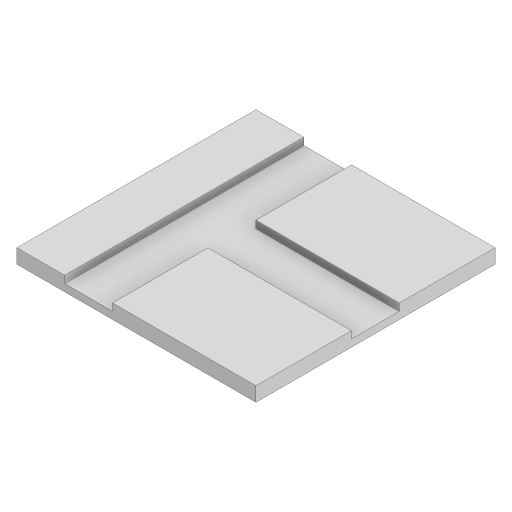
# Autodesk Inventor part: T_intersection_simple
Saved by Autodesk Inventor 2023 (Build 270158000, 158)
## iProperties
Created: 2022-07-19
Part Number: T_intersection_simple
Material: Generic
Document SubType Name: Modeling
Designer: Derm
Density: 1 g/cm^3
Appearance: Default
Author: Derm
Autodesk Inventor part; units mm, degrees
ref_plane "YZ Plane" through (0, 0, 0) normal (1, 0, 0) x (0, 1, 0)
ref_plane "XZ Plane" through (0, 0, 0) normal (0, 1, 0) x (-1, 0, 0)
ref_plane "XY Plane" through (0, 0, 0) normal (0, 0, 1) x (1, 0, 0)
sketch "Sketch1" plane through (0, 0, 0) normal (0, 1, 0) x (-1, 0, 0)
  line L0 (-50000, 50000) -> (50000, 50000)
  line L1 (50000, 50000) -> (50000, -50000)
  line L2 (50000, -50000) -> (-50000, -50000)
  line L3 (-50000, -50000) -> (-50000, 50000)
  line L4 (-50000, 50000) -> (50000, -50000) construction
  line L5 (50000, 50000) -> (-50000, -50000) construction
  point P0 (0, 0)
  dimension "d0" = 100000
  dimension "d1" = 100000
  constraints: 12 end point, 2 midpoint, 2 parallel, 1 horizontal, 1 perpendicular
  measures "d0" distance of L1.end L2.end
  measures "d1" distance of L0.end L1.end
extrude "Extrusion1" add sketch "Sketch1" against normal blind 3000
sketch "Sketch2" plane through (0, 0, 0) normal (0, 1, 0) x (1, 0, 0)
  line L0 (50000, 50000) -> (-50000, 50000) projected
  line L1 (-50000, 50000) -> (-50000, -50000) projected
  line L2 (-50000, -50000) -> (50000, -50000) projected
  line L3 (50000, -50000) -> (50000, 50000) projected
  line L4 (50000, 50000) -> (50000, -50000) projected
  line L5 (50000, -50000) -> (-10000, -50000)
  line L6 (-10000, -50000) -> (-10000, -10100.7954)
  line L7 (-10000, -10100.7954) -> (50000, -10100.7954)
  line L8 (50000, -10100.7954) -> (50000, -50000)
  line L9 (-50000, 50000) -> (50000, 50000) projected
  line L10 (50000, 50000) -> (-10000, 50000)
  line L11 (-10000, 50000) -> (-10000, 9899.2046)
  line L12 (-10000, 9899.2046) -> (50000, 9899.2046)
  line L13 (50000, 9899.2046) -> (50000, 50000)
  line L14 (-50000, -50000) -> (-30000, -50000)
  line L15 (-30000, -50000) -> (-30000, 50000)
  line L16 (-30000, 50000) -> (-50000, 50000)
  line L17 (-50000, 50000) -> (-50000, -50000)
  point P0 (0, 0)
  point P1 (50000, 9899.2046)
  point P2 (-30000, -50000)
  point P3 (50000, -10100.7954)
  point P4 (-10000, -50000)
  dimension "d4" = 60000
  dimension "d5" = 20000
  dimension "d6" = 20000
  constraints: 24 end point, 6 parallel, 3 horizontal, 3 perpendicular, 2 point on line
  measures "d4" distance between parallel lines of L3 L6
  measures "d5" distance between parallel lines of L12 L7
  measures "d6" distance between parallel lines of L6 L15
extrude "Extrusion2" add sketch "Sketch2" along normal blind 3000 contours L3 L12 L11 L0 | L15 L2 L1 L0 | L3 L2 L6 L7
body "Solid1"
